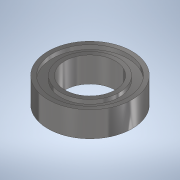
# Autodesk Inventor part: ベアリングHd6-D10-B3F無し甲
Saved by Autodesk Inventor 2020.2 (Build 242310000, 310)
## iProperties
Created: 2017-02-12
Part Number: ベアリングHd6-D10-B3F無し甲
Material: 鋼、炭素鋼
Document SubType Name: Modeling
Designer: 大空
Mass: 0.77 g
Surface Area: 3.43816 cm^2
Volume: 0.137652 cm^3
Density: 7.85 g/cm^3
Appearance: 半つや出し
Author: 大空
Autodesk Inventor part; units mm, degrees
ref_plane "YZ Plane" through (0, 0, 0) normal (1, 0, 0) x (0, 1, 0)
ref_plane "XZ Plane" through (0, 0, 0) normal (0, 1, 0) x (-1, 0, 0)
ref_plane "XY Plane" through (0, 0, 0) normal (0, 0, 1) x (1, 0, 0)
sketch "スケッチ1" plane through (0, 0, 0) normal (0, 0, 1) x (1, 0, 0)
  circle A0 centre (0, 0) radius 3
  circle A1 centre (0, 0) radius 5
  dimension "d0" = 6
  dimension "d1" = 10
  constraints: 2 centre point, 2 coincident
  measures "d0" diameter of A0
  measures "d1" diameter of A1
extrude "押し出し1" add sketch "スケッチ1" along normal blind 3
sketch "スケッチ2" plane through (0, 0, 0) normal (0, 0, -1) x (-1, 0, 0)
  circle A0 centre (0, 0) radius 3 projected
  circle A1 centre (0, 0) radius 5 projected
  circle A2 centre (0, 0) radius 5.6
  dimension "d4" = 11.2
  constraints: 1 centre point, 1 coincident
  measures "d4" diameter of A2
extrude "押し出し2" add sketch "スケッチ2" against normal blind 0.6 contours A2
sketch "スケッチ3" plane through (0, 0, 3) normal (0, 0, 1) x (1, 0, 0)
  circle A0 centre (0, 0) radius 3 projected
  circle A1 centre (0, 0) radius 5 projected
  circle A2 centre (0, 0) radius 4.5
  circle A3 centre (0, 0) radius 3.5
  dimension "d7" = 0.5
  dimension "d8" = 0.5
  constraints: 2 centre point
  measures "d7" radial gap between concentric circles of A1 A2
  measures "d8" radial gap between concentric circles of A0 A3
extrude "押し出し3" cut sketch "スケッチ3" against normal blind 0.5 contours A2
sketch "スケッチ4" plane through (0, 0, 0) normal (0, 0, -1) x (-1, 0, 0)
  circle A0 centre (0, 0) radius 3.5 projected
  circle A1 centre (0, 0) radius 4.5 projected
extrude "押し出し4" cut sketch "スケッチ4" against normal blind 0.5
sketch "スケッチ5" plane through (0, 0, 0) normal (0, 0, -1) x (-1, 0, 0)
  point P0 (0, 0)
sketch "スケッチ6" plane through (0, 0, 0.6) normal (0, 0, 1) x (1, 0, 0)
  circle A0 centre (0, 0) radius 5
  circle A1 centre (0, 0) radius 5.6
  dimension "d13" = 10
  dimension "d14" = 0.6
  constraints: 2 centre point, 1 coincident
  measures "d13" diameter of A0
  measures "d14" radial gap between concentric circles of A0 A1
extrude "押し出し5" cut sketch "スケッチ6" against normal blind 0.6
